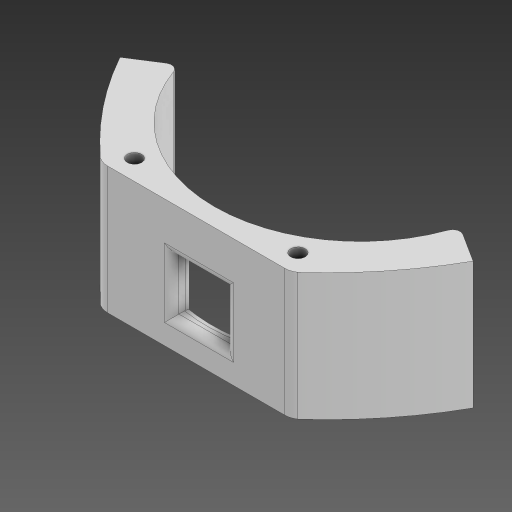
# Autodesk Inventor part: ball_solenoid_v2
Saved by Autodesk Inventor 2023 (Build 270158000, 158)
## iProperties
Created: 2025-06-23
Part Number: ball_solenoid_v2
Material: Типовые
Document SubType Name: Modeling
Designer: daa
Density: 1 g/cm^3
Appearance: По умолчанию
Author: daa
Autodesk Inventor part; units mm, degrees
ref_plane "YZ Plane" through (0, 0, 0) normal (1, 0, 0) x (0, 1, 0)
ref_plane "XZ Plane" through (0, 0, 0) normal (0, 1, 0) x (-1, 0, 0)
ref_plane "XY Plane" through (0, 0, 0) normal (0, 0, 1) x (1, 0, 0)
sketch "Эскиз1" plane through (0, 0, 0) normal (0, 1, 0) x (-1, 0, 0)
  line L0 (-24.3583, 67.9739) -> (24.3787, 67.9739)
  arc A0 (38.6021, 33.9735) -> (-38.5819, 33.9735) centre (0.0101, 22.7957) ccw
  arc A1 (36.6633, -21.4663) -> (-36.0003, -21.4663) centre (0.3315, -28.4663) ccw
  line L1 (36.6633, -21.4663) -> (-36.0003, -21.4663)
  circle A2 centre (22.5101, 62.4739) radius 2
  circle A3 centre (-22.4899, 62.4739) radius 2
  arc A4 (27.1475, 67.1373) -> (24.3787, 67.9739) centre (24.3787, 62.9739) ccw
  arc A5 (-24.3583, 67.9739) -> (-27.1271, 67.1373) centre (-24.3583, 62.9739) ccw
  line L2 (38.6021, 33.9735) -> (-38.5819, 33.9735)
  line L3 (38.6021, 33.9735) -> (48.6021, 33.9735)
  line L4 (38.6021, 33.9735) -> (48.6021, 40.351)
  line L5 (-38.5819, 33.9735) -> (-48.5819, 33.9735)
  line L6 (-38.5819, 33.9735) -> (-48.5819, 40.351)
  arc A6 (48.6021, 40.351) -> (27.1475, 67.1373) centre (-42.1852, -10.3804) ccw
  arc A7 (-27.1271, 67.1373) -> (-48.5819, 40.351) centre (42.2052, -10.3807) ccw
  point P0 (0, 0)
  point P1 (0, 0)
  point P2 (-25.8456, 67.9739)
  point P3 (0.0102, 67.9739)
  point P4 (0, 0)
  point P5 (25.866, 67.9739)
  point P6 (-25.8046, 67.7601)
  point P7 (25.8249, 67.7602)
  point P8 (0.0101, 62.9739)
  point P9 (0.0101, 33.9735)
  dimension "d0" = 72.6636
  dimension "d1" = 37
  dimension "d4" = 5.5
  dimension "d5" = 5.5
  dimension "d8" = 5
  dimension "d105" = 77.184
  dimension "d108" = 4
  dimension "d109" = 4
  dimension "d111" = 40.1782
  dimension "d112" = 5
  dimension "d113" = 10
  dimension "d114" = 10
  dimension "d115" = 10
  dimension "d117" = 104
  dimension "d118" = 104
  dimension "d135" = 45
  dimension "d136" = 48.737
  dimension "d140" = 22.5
  constraints: 15 point on circle, 14 end point, 8 centre point, 5 horizontal, 2 midpoint, 2 point on line, 2 tangent, 1 equal radius
  measures "d0" distance of L1.start L1.end
  measures "d1" radius of A1
  measures "d4" vertical distance of point (25.866, 67.974) A2.centre
  measures "d5" vertical distance of point (-25.846, 67.974) A3.centre
  measures "d8" radius of A4
  measures "d105" distance of L2.end L2.start
  measures "d108" diameter of A2
  measures "d109" diameter of A3
  measures "d111" radius of A0
  measures "d112" distance of point (0.01, 67.974) point (0.01, 62.974)
  measures "d113" distance of L2.start L3.end
  measures "d114" horizontal distance of L2.start L4.end
  measures "d115" distance of L2.end L5.end
  measures "d117" radius of A6
  measures "d118" radius of A7
  measures "d135" distance of A2.centre A3.centre
  measures "d136" distance of L0.start L0.end
  measures "d140" horizontal distance of A3.centre point (0.01, 62.974)
extrude "Выдавливание1" add sketch "Эскиз1" along normal blind 35 contours L0 A4 A6 L4 A0 L6 A7 A5
sketch "Эскиз7" plane through (-24.3787, 0, 67.9739) normal (0, 0, 1) x (1, 0, 0)
  line L0 (17.61, 22.5) -> (32.61, 22.5)
  line L1 (32.61, 22.5) -> (32.61, 7.5)
  line L2 (32.61, 7.5) -> (17.61, 7.5)
  line L3 (17.61, 7.5) -> (17.61, 22.5)
  line L4 (0, 35) -> (48.737, 35) projected
  line L5 (0, 0) -> (0, 35) projected
  point P0 (24.3787, 0)
  dimension "d40" = 15
  dimension "d41" = 15
  dimension "d42" = 12.5
  dimension "d43" = 17.61
  constraints: 8 end point, 2 parallel, 1 horizontal, 1 perpendicular
  measures "d40" distance of L1.end L2.end
  measures "d41" distance of L0.end L1.end
  measures "d42" distance between parallel lines of L4 L0
  measures "d43" distance between parallel lines of L5 L3
extrude "Выдавливание5" cut sketch "Эскиз7" against normal blind 48
fillet "Сопряжение1" radius 2 8 edges at (0.7313, 7.5, 67.9739) (-6.7687, 15, 67.9739) (0.7313, 22.5, 67.9739) (8.2313, 15, 67.9739) (8.2313, 15, 62.1195) (0.7446, 22.5, 62.9668) (-6.7687, 15, 62.4013) (0.7446, 7.5, 62.9668)
fillet "Сопряжение2" radius 2 2 edges at (38.5819, 17.5, 33.9735) (-38.6021, 17.5, 33.9735)
sketch "Эскиз18" plane through (48.5819, 0, 40.351) normal (0.5377055, 0, -0.8431327) x (-0.8431327, 0, -0.5377055)
  circle A0 centre (5.5955, 27.5) radius 2
  circle A1 centre (5.5955, 7.5) radius 2
  line L0 (0, 35) -> (9.275, 35) projected
  line L1 (11.2255, 0) -> (11.2255, 35) projected
  point P0 (62.658, 0)
  dimension "d119" = 4
  dimension "d120" = 4
  dimension "d121" = 20
  dimension "d122" = 7.5
  dimension "d123" = 5.63
  dimension "d124" = 5.63
  constraints: 2 centre point
  measures "d119" diameter of A0
  measures "d120" diameter of A1
  measures "d121" distance of A1.centre A0.centre
  measures "d122" distance from line of L0 A0.centre
  measures "d123" distance from line of L1 A0.centre
  measures "d124" distance from line of L1 A1.centre
extrude "Выдавливание12" cut sketch "Эскиз18" against normal blind 5
sketch "Эскиз20" plane through (-48.6021, 0, 40.351) normal (-0.5377055, 0, -0.8431327) x (-0.8431327, 0, 0.5377055)
  circle A0 centre (-5.63, 27.5) radius 2
  circle A1 centre (-5.63, 7.5) radius 2
  line L0 (-9.275, 35) -> (0, 35) projected
  line L1 (0, 0) -> (0, 35) projected
  point P0 (-62.675, 0)
  point P1 (-4.6375, 35)
  dimension "d127" = 4
  dimension "d128" = 4
  dimension "d129" = 20
  dimension "d130" = 7.5
  dimension "d131" = 5.63
  dimension "d132" = 5.63
  constraints: 2 centre point, 1 midpoint
  measures "d127" diameter of A0
  measures "d128" diameter of A1
  measures "d129" distance of A1.centre A0.centre
  measures "d130" vertical distance of point (-4.638, 35) A0.centre
  measures "d131" distance from line of L1 A0.centre
  measures "d132" distance from line of L1 A1.centre
extrude "Выдавливание13" cut sketch "Эскиз20" against normal blind 5
